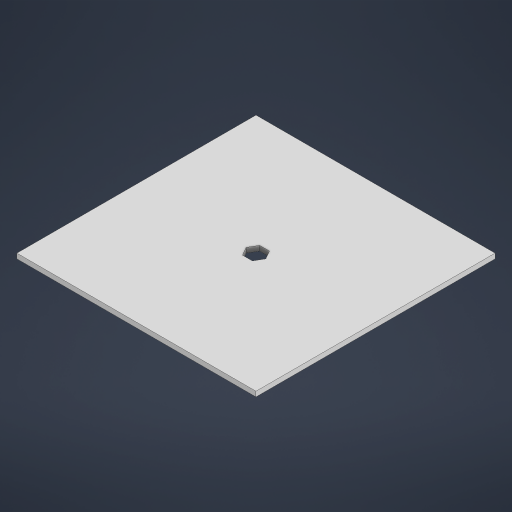
# Autodesk Inventor part: TurretGear
Saved by Autodesk Inventor 2023 (Build 270158000, 158)
## iProperties
Created: 2022-04-16
Part Number: TurretGear
Material: Generic
Document SubType Name: Modeling
Designer: timmy
Density: 1 g/cm^3
Appearance: Default
Author: timmy
Autodesk Inventor part; units mm, degrees
ref_plane "YZ Plane" through (0, 0, 0) normal (1, 0, 0) x (0, 1, 0)
ref_plane "XZ Plane" through (0, 0, 0) normal (0, 1, 0) x (-1, 0, 0)
ref_plane "XY Plane" through (0, 0, 0) normal (0, 0, 1) x (1, 0, 0)
sketch "Sketch1" plane through (0, 0, 0) normal (0, 1, 0) x (-1, 0, 0)
  circle A0 centre (0, 0) radius 76.2
  line L0 (-77.0001, 77.0001) -> (77.0001, 77.0001)
  line L1 (77.0001, 77.0001) -> (77.0001, -77.0001)
  line L2 (77.0001, -77.0001) -> (-77.0001, -77.0001)
  line L3 (-77.0001, -77.0001) -> (-77.0001, 77.0001)
  line L4 (-77.0001, 77.0001) -> (77.0001, -77.0001) construction
  line L5 (77.0001, 77.0001) -> (-77.0001, -77.0001) construction
  dimension "d0" = 152.4
  dimension "d7" = 154.0002
  dimension "d8" = 154.0002
  constraints: 12 end point, 2 midpoint, 2 parallel, 1 centre point, 1 coincident, 1 horizontal, 1 perpendicular
  measures "d0" diameter of A0
  measures "d7" distance of L1.end L2.end
  measures "d8" distance of L0.end L1.end
extrude "Extrusion1" add sketch "Sketch1" along normal blind 3.175 contours A0 | L0 L1 L2 L3
sketch "Sketch2" plane through (0, 3.175, 0) normal (0, 1, 0) x (1, 0, 0)
  line L0 (0, 0) -> (-6.35, 0)
  line L1 (-6.35, 0) -> (-3.175, 5.4993)
  line L2 (-3.175, 5.4993) -> (3.175, 5.4993)
  line L3 (3.175, 5.4993) -> (6.35, 0)
  line L4 (6.35, 0) -> (3.175, -5.4993)
  line L5 (3.175, -5.4993) -> (-3.175, -5.4993)
  line L6 (-3.175, -5.4993) -> (-6.35, 0)
  dimension "d4" = 6.35
  constraints: 14 end point, 1 coincident, 1 horizontal, 13 other
  measures "d4" distance of L0.start L0.end
extrude "Extrusion2" cut sketch "Sketch2" against normal blind 3.175
body "Solid1"
